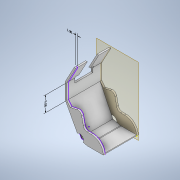
# Autodesk Inventor part: Seat
Saved by Autodesk Inventor 2021 (Build 250183000, 183)
## iProperties
Created: 2020-10-04
Part Number: Seat
Material: Generic
Document SubType Name: Modeling
Designer: PhotonUser
Density: 1 g/cm^3
Appearance: Default
Author: PhotonUser
Autodesk Inventor part; units mm, degrees
ref_plane "YZ Plane" through (0, 0, 0) normal (1, 0, 0) x (0, 1, 0)
ref_plane "XZ Plane" through (0, 0, 0) normal (0, 1, 0) x (-1, 0, 0)
sketch "Sketch1" plane through (0, 0, 0) normal (0, 0, 1) x (1, 0, 0)
  line L0 (0, 0) -> (-241.3, 0)
  line L1 (-352.8762, 28.575) -> (-241.3, 0)
  line L2 (-568.379, 431.8) -> (-352.8762, 28.575)
  arc A0 (-1.9317, 0) -> (-179.7317, 177.8) centre (-179.7317, 0) ccw
  arc A1 (-321.8515, 344.496) -> (-394.4455, 390.1126) centre (-380.6333, 331.522) ccw
  line L3 (-179.7317, 177.8) -> (-238.6526, 177.8)
  line L4 (-321.8515, 344.496) -> (-296.6352, 230.2477)
  arc A2 (-296.6352, 230.2477) -> (-238.6526, 177.8) centre (-238.6526, 236.0747) ccw
  line L5 (-490.4406, 367.4826) -> (-394.4455, 390.1126)
  line L6 (-568.379, 431.8) -> (-568.379, 660.4)
  line L7 (-542.979, 660.4) -> (-542.979, 431.8)
  line L8 (-542.979, 431.8) -> (-490.4406, 367.4826)
  line L9 (-431.7117, 914.4) -> (-568.379, 660.4)
  line L10 (-406.3016, 914.4) -> (-542.979, 660.4)
  line L11 (-406.3016, 914.4) -> (-431.7117, 914.4)
  constraints: 24 end point, 6 point on circle, 3 centre point, 3 horizontal, 3 point on line, 2 tangent, 1 vertical
sketch "Sketch4" plane through (0, 0, 0) normal (0, 0, 1) x (1, 0, 0)
  line L0 (0, 0) -> (-241.3, 0)
  line L1 (-352.8762, 28.575) -> (-241.3, 0)
  line L2 (-568.379, 431.8) -> (-352.8762, 28.575)
  line L3 (-568.379, 431.8) -> (-568.379, 660.4)
  line L4 (-542.979, 660.4) -> (-542.979, 431.8)
  line L5 (-431.7117, 914.4) -> (-568.379, 660.4)
  line L6 (-406.3016, 914.4) -> (-542.979, 660.4)
  line L7 (-406.3016, 914.4) -> (-431.7117, 914.4)
  line L8 (-1.9317, 0) -> (-2.3853, 12.6919)
  line L9 (-241.3, 0) -> (-228.6, 0)
  line L10 (-228.6, 0) -> (-228.6, 12.7)
  line L11 (-2.3853, 12.6919) -> (-228.6, 12.7)
  line L12 (-228.6, 12.7) -> (-290.8894, 12.7)
  line L13 (-241.3, 0) -> (-241.3, 12.7)
  line L14 (-352.8762, 28.575) -> (-352.8762, 41.275)
  line L15 (-352.8762, 41.275) -> (-241.3, 12.7)
  line L16 (-352.8762, 41.275) -> (-542.979, 431.8)
  dimension "d63" = 12.7
  dimension "d64" = 12.7
  dimension "d65" = 12.7
  dimension "d66" = 12.7
  dimension "d68" = 12.7
  constraints: 34 end point, 5 point on line, 3 horizontal, 3 vertical
  measures "d63" distance of L8.start L8.end
  measures "d64" distance of L0.end L9.end
  measures "d65" distance of L9.end L10.end
  measures "d66" distance of L0.end L13.end
  measures "d68" distance of L1.start L14.end
extrude "Extrusion1" add sketch "Sketch4" against normal blind 469.9
extrude "Extrusion2" add sketch "Sketch1" along normal blind 25.4
ref_plane "Work Plane3" through (0, 0, -469.9) normal (0, 0, 1) x (1, 0, 0)
sketch "Sketch5" plane through (0, 0, 0) normal (0, 0, 1) x (1, 0, 0)
  line L0 (0, 0) -> (-241.3, 0)
  line L1 (-352.8762, 28.575) -> (-241.3, 0)
  line L2 (-568.379, 431.8) -> (-352.8762, 28.575)
  arc A0 (-1.9317, 0) -> (-179.7317, 177.8) centre (-179.7317, 0) ccw
  arc A1 (-321.8515, 344.496) -> (-394.4455, 390.1126) centre (-380.6333, 331.522) ccw
  line L3 (-179.7317, 177.8) -> (-238.6526, 177.8)
  line L4 (-321.8515, 344.496) -> (-296.6352, 230.2477)
  arc A2 (-296.6352, 230.2477) -> (-238.6526, 177.8) centre (-238.6526, 236.0747) ccw
  line L5 (-490.4406, 367.4826) -> (-394.4455, 390.1126)
  line L6 (-568.379, 431.8) -> (-568.379, 660.4)
  line L7 (-542.979, 660.4) -> (-542.979, 431.8)
  line L8 (-542.979, 431.8) -> (-490.4406, 367.4826)
  line L9 (-431.7117, 914.4) -> (-568.379, 660.4)
  line L10 (-406.3016, 914.4) -> (-542.979, 660.4)
  line L11 (-406.3016, 914.4) -> (-431.7117, 914.4)
  constraints: 24 end point, 6 point on circle, 3 centre point, 3 horizontal, 3 point on line, 2 tangent, 1 vertical
sketch "Sketch6" plane through (0, 0, -469.9) normal (0, 0, 1) x (1, 0, 0)
  point P0 (0, 0)
sketch "Sketch7" plane through (0, 0, -469.9) normal (0, 0, 1) x (1, 0, 0)
  line L0 (0, 0) -> (-241.3, 0)
  line L1 (-352.8762, 28.575) -> (-241.3, 0)
  line L2 (-568.379, 431.8) -> (-352.8762, 28.575)
  arc A0 (-1.9317, 0) -> (-179.7317, 177.8) centre (-179.7317, 0) ccw
  arc A1 (-321.8515, 344.496) -> (-394.4455, 390.1126) centre (-380.6333, 331.522) ccw
  line L3 (-179.7317, 177.8) -> (-238.6526, 177.8)
  line L4 (-321.8515, 344.496) -> (-296.6352, 230.2477)
  arc A2 (-296.6352, 230.2477) -> (-238.6526, 177.8) centre (-238.6526, 236.0747) ccw
  line L5 (-490.4406, 367.4826) -> (-394.4455, 390.1126)
  line L6 (-568.379, 431.8) -> (-568.379, 660.4)
  line L7 (-542.979, 660.4) -> (-542.979, 431.8)
  line L8 (-542.979, 431.8) -> (-490.4406, 367.4826)
  line L9 (-431.7117, 914.4) -> (-568.379, 660.4)
  line L10 (-406.3016, 914.4) -> (-542.979, 660.4)
  line L11 (-406.3016, 914.4) -> (-431.7117, 914.4)
  constraints: 24 end point, 6 point on circle, 3 centre point, 3 horizontal, 3 point on line, 2 tangent, 1 vertical
extrude "Extrusion3" add sketch "Sketch7" against normal blind 25.4
sketch "Sketch8" plane through (0, 0, 0) normal (1, 0, 0) x (0, 1, 0)
  line L0 (0, 0) -> (0, -228.6)
  line L1 (0, -495.3) -> (0, 25.4) projected
  line L2 (0, -228.6) -> (596.9, -228.6)
  line L3 (660.4, -495.3) -> (660.4, 25.4) projected
  line L4 (596.9, -228.6) -> (596.9, -95.25)
  line L5 (431.8, 0) -> (431.8, -469.9) projected
  line L6 (596.9, -228.6) -> (596.9, -361.95)
  line L7 (596.9, -361.95) -> (1104.9, -361.95)
  line L8 (1104.9, -361.95) -> (1104.9, -95.25)
  line L9 (1104.9, -95.25) -> (596.9, -95.25)
  line L10 (596.9, -95.25) -> (660.4, -95.25)
  line L11 (660.4, -95.25) -> (685.8, -95.25)
  line L12 (685.8, -95.25) -> (685.8, -142.875)
  line L13 (685.8, -142.875) -> (1104.9, -142.875)
  line L14 (660.4, -361.95) -> (685.8, -361.95)
  line L15 (685.8, -361.95) -> (685.8, -314.325)
  line L16 (685.8, -314.325) -> (1104.9, -314.325)
  dimension "d77" = 228.6
  dimension "d78" = 596.9
  dimension "d80" = 133.35
  dimension "d81" = 133.35
  dimension "d82" = 508
  dimension "d83" = 266.7
  dimension "d84" = 25.4
  dimension "d85" = 47.625
  dimension "d86" = 47.625
  constraints: 28 end point, 9 point on line, 6 perpendicular, 2 vertical, 1 parallel
  measures "d77" distance of L0.start L0.end
  measures "d78" distance of L0.end L2.end
  measures "d80" distance of L2.end L4.end
  measures "d81" distance of L2.end L6.end
  measures "d82" distance of L6.end L7.end
  measures "d83" distance of L7.end L8.end
  measures "d84" distance of L10.end L11.end
  measures "d85" distance of L11.end L12.end
  measures "d86" distance of L14.end L15.end
extrude "Extrusion4" cut sketch "Sketch8" against normal blind 914.4 contours L7 L6 L4 L9 L3 | L3 L9 L12 L13 L8 L16 L15 L7
sketch "Sketch11" plane through (0, 0, -495.3) normal (0, 0, -1) x (-1, 0, 0)
  line L0 (352.8762, 28.575) -> (241.3, 0) projected
  circle A0 centre (352.8762, 28.575) radius 60.325
  point P0 (0, 0)
  dimension "d92" = 120.65
  constraints: 1 centre point
  measures "d92" diameter of A0
extrude "Extrusion6" cut sketch "Sketch11" against normal blind 25.4
sketch "Sketch12" plane through (0, 0, 25.4) normal (0, 0, 1) x (1, 0, 0)
  line L0 (-241.3, 12.7) -> (-352.8762, 41.275) projected
  circle A0 centre (-352.8762, 41.275) radius 60.325
  point P0 (0, 0)
  dimension "d95" = 120.65
  constraints: 1 centre point
  measures "d95" diameter of A0
extrude "Extrusion7" cut sketch "Sketch12" against normal blind 25.4
equation "\"SeatBottomDepth\" = 241.3"
equation "\"SeatFrontBottomWidth\" = 469.9"
equation "\"SeatFrontSidesWidth\" = 520.7"
equation "\"SeatBackInnerWidth\" = 304.8"
equation "\"SeatBackOuterWidth\" = 482.6"
equation "\"SeatBackLength\" = 457.2"
body "Solid1"
